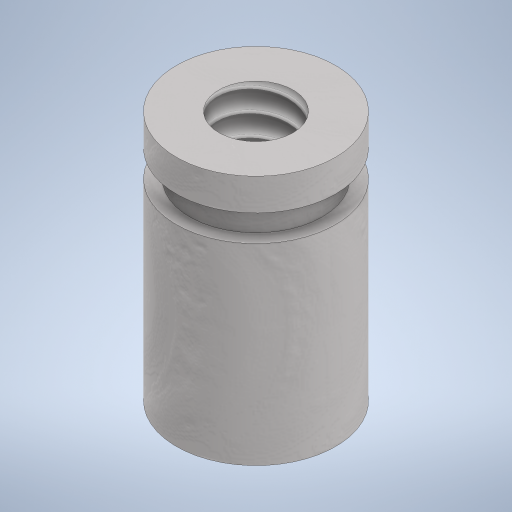
# Autodesk Inventor part: Guia do eixo roscado
Saved by Autodesk Inventor 2023 (Build 270158000, 158)
## iProperties
Created: 2023-03-22
Part Number: Guia do eixo roscado
Material: Aço
Document SubType Name: Sheet Metal
Designer: Mateus
Density: 7.85 g/cm^3
Sheet Metal Rule: Default_mm
Appearance: Aço suave - Soldado
Mass: 212.855 g
Surface Area: 77.5581 cm^2
Volume: 27.1153 cm^3
Author: Mateus
Autodesk Inventor part; units mm, degrees
ref_plane "YZ Plane" through (0, 0, 0) normal (1, 0, 0) x (0, 1, 0)
ref_plane "XZ Plane" through (0, 0, 0) normal (0, 1, 0) x (-1, 0, 0)
ref_plane "XY Plane" through (0, 0, 0) normal (0, 0, 1) x (1, 0, 0)
sketch "Esboço1" plane through (0, 0, 0) normal (0, 1, 0) x (-1, 0, 0)
  circle A0 centre (0, 0) radius 15
  dimension "d0" = 30
  constraints: 1 centre point, 1 coincident
  measures "d0" diameter of A0
extrude "Extrusão1" add sketch "Esboço1" along normal blind 36.24
sketch "Esboço2" plane through (0, 36.24, 0) normal (0, 1, 0) x (1, 0, 0)
  circle A0 centre (0, 0) radius 12.5
  dimension "d3" = 25
  constraints: 1 centre point, 1 coincident
  measures "d3" diameter of A0
extrude "Extrusão2" add sketch "Esboço2" along normal blind 5
sketch "Esboço3" plane through (0, 41.24, 0) normal (0, 1, 0) x (1, 0, 0)
  circle A0 centre (0, 0) radius 15
  constraints: 1 centre point, 1 coincident
extrude "Extrusão3" add sketch "Esboço3" along normal blind 6
sketch "Sketch5" plane through (0, 47.24, 0) normal (0, 1, 0) x (1, 0, 0)
  circle A0 centre (0, 0) radius 15 projected
  constraints: 1 coincident
hole "Hole2" at (0, 47.24, 0) direction (0, -1, 0) diameter 14 end through all
thread "Thread1" size "M52x4" class "6H" standard "ANSI Metric M Profile" full length
equation "\"d20\" = Espessura"
equation "\"Raio_vergadura\" = Espessura"
equation "\"Largura_alívio_de_vergadura\" = Espessura"
equation "\"Profundidade_alívio_de_vergadura\" = 0.5 * Espessura"
equation "\"Tamanho_alívio_de_dobra\" = 4 * Espessura"
equation "\"Remanescente_mínimo\" = 2 * Espessura"
equation "\"Raiodetransição\" = Raio_vergadura"
equation "\"Tamanho_de_raio_de_Jacobi\" = Raio_vergadura"
equation "\"TamanhoFolga\" = Espessura"
equation "\"Espessura\" = 0.5"
